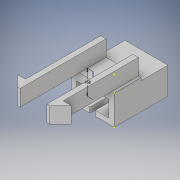
# Autodesk Inventor part: Small USB Cover
Saved by Autodesk Inventor 2018 (Build 220112000, 112)
## iProperties
Created: 2018-01-13
Part Number: Small USB Cover
Material: Generic
Document SubType Name: Modeling
Designer: cruz.anthony
Density: 1 g/cm^3
Appearance: Default
Author: cruz.anthony
Autodesk Inventor part; units mm, degrees
ref_plane "YZ Plane" through (0, 0, 0) normal (1, 0, 0) x (0, 1, 0)
ref_plane "XZ Plane" through (0, 0, 0) normal (0, 1, 0) x (-1, 0, 0)
ref_plane "XY Plane" through (0, 0, 0) normal (0, 0, 1) x (1, 0, 0)
sketch "Sketch1" plane through (0, 0, 0) normal (0, 1, 0) x (-1, 0, 0)
  line L0 (0, 0) -> (20.32, 0)
  line L1 (20.32, 0) -> (20.32, -27.94)
  line L2 (20.32, -27.94) -> (0, -27.94)
  line L3 (0, -27.94) -> (0, 0)
  dimension "d0" = 20.32
  dimension "d1" = 27.94
  constraints: 8 end point, 2 parallel, 1 horizontal, 1 perpendicular
  measures "d0" distance of L1.end L2.end
  measures "d1" distance of L0.end L1.end
extrude "Extrusion1" add sketch "Sketch1" along normal blind 12.7
sketch "Sketch2" plane through (-20.32, 0, 0) normal (0, 0, 1) x (1, 0, 0)
  line L0 (2.54, 2.54) -> (17.78, 2.54)
  line L1 (17.78, 2.54) -> (17.78, 10.16)
  line L2 (17.78, 10.16) -> (2.54, 10.16)
  line L3 (2.54, 10.16) -> (2.54, 2.54)
  point P0 (0, 0)
  dimension "d6" = 15.24
  dimension "d7" = 7.62
  constraints: 8 end point, 2 parallel, 1 horizontal, 1 perpendicular
  measures "d6" distance of L2.end L1.end
  measures "d7" distance of L1.end L0.end
extrude "Extrusion2" cut sketch "Sketch2" against normal blind 22.86
sketch "Sketch3" plane through (0, 0, -27.94) normal (0, 0, -1) x (-1, 0, 0)
  line L0 (0, 0) -> (0, 12.7) projected
  line L1 (0, 0) -> (20.32, 0) projected
  line L2 (0, 12.7) -> (20.32, 12.7)
  line L3 (20.32, 12.7) -> (20.32, 0)
  line L4 (20.32, 0) -> (0, 0)
  line L5 (0, 0) -> (0, 12.7)
  constraints: 8 end point, 2 parallel, 1 horizontal, 1 perpendicular
extrude "Extrusion3" cut sketch "Sketch3" against normal blind 2.54
sketch "Sketch4" plane through (0, 0, 0) normal (0, -1, 0) x (1, 0, 0)
  line L0 (-8.89, 0) -> (-11.43, 0)
  line L1 (-11.43, 0) -> (-11.43, -25.4)
  line L2 (-11.43, -25.4) -> (-8.89, -25.4)
  line L3 (-8.89, -25.4) -> (-8.89, 0)
  line L4 (-20.32, 0) -> (-20.32, -25.4) projected
  line L5 (0, -25.4) -> (0, 0) projected
  dimension "d12" = 8.89
  dimension "d32" = 8.89
  constraints: 8 end point, 2 parallel, 1 horizontal, 1 perpendicular
  measures "d12" distance of L5.end L0.start
  measures "d32" distance between parallel lines of L4 L1
sketch "Sketch5" plane through (0, 0, -25.4) normal (0, 0, -1) x (-1, 0, 0)
  line L0 (0, 0) -> (20.32, 0) projected
  line L1 (10.16, 0) -> (10.16, 6.35)
  circle A0 centre (10.16, 6.35) radius 1.27
  dimension "d14" = 6.35
  dimension "d15" = 2.54
  constraints: 2 end point, 1 centre point, 1 coincident, 1 midpoint, 1 vertical
  measures "d14" distance of L1.start L1.end
  measures "d15" diameter of A0
extrude "Extrusion4" cut sketch "Sketch5" against normal blind 2.54
extrude "Extrusion5" cut sketch "Sketch4" against normal blind 6.35
sketch "Sketch8" plane through (0, 12.7, 0) normal (0, 1, 0) x (1, 0, 0)
  line L0 (0, 25.4) -> (0, 0) projected
  line L1 (-20.32, 0) -> (-20.32, 25.4) projected
  line L2 (0, 0) -> (-20.32, 0)
  line L3 (-20.32, 0) -> (-20.32, 12.7)
  line L4 (-20.32, 12.7) -> (0, 12.7)
  line L5 (0, 12.7) -> (0, 0)
  constraints: 8 end point, 2 parallel, 1 horizontal, 1 midpoint, 1 perpendicular
extrude "Extrusion8" add sketch "Sketch8" along normal blind 2.54
sketch "Sketch9" plane through (-17.78, 10.16, 0) normal (0, 0, 1) x (1, 0, 0)
  arc A0 (8.89, -3.81) -> (6.35, -3.81) centre (7.62, -3.81) ccw projected
  line L0 (7.62, -3.81) -> (7.62, 7.62)
  point P0 (17.78, -10.16)
  dimension "d36" = 11.43
  constraints: 2 end point, 1 vertical
  measures "d36" distance of L0.start L0.end
sketch "Sketch10" plane through (0, 15.24, 0) normal (0, 1, 0) x (1, 0, 0)
  line L0 (-11.43, 0) -> (-20.32, 0) projected
  line L1 (-20.32, 0) -> (0, 0)
  line L2 (0, 0) -> (0, 12.7)
  line L3 (0, 12.7) -> (-20.32, 12.7)
  line L4 (-20.32, 12.7) -> (-20.32, 0)
  constraints: 8 end point, 2 parallel, 1 horizontal, 1 perpendicular
extrude "Extrusion9" cut sketch "Sketch10" against normal blind 1.27
sketch "Sketch11" plane through (0, 13.97, 0) normal (0, 1, 0) x (1, 0, 0)
  point P0 (0, 0)
sketch "Sketch12" plane through (0, 13.97, 0) normal (0, 1, 0) x (1, 0, 0)
  line L0 (-17.78, 0) -> (-2.54, 0) projected
  line L1 (-10.16, 0) -> (-10.16, 12.7099)
  line L2 (-10.16, 0) -> (-16.51, 0)
  line L3 (-11.43, 0) -> (-20.32, 0) projected
  line L4 (-10.16, 0) -> (-3.81, 0)
  line L5 (-3.81, 0) -> (0, 0)
  line L6 (0, 0) -> (0, 12.7099)
  line L7 (0, 12.7099) -> (-3.81, 12.7099)
  line L8 (-3.81, 12.7099) -> (-3.81, 0)
  line L9 (-20.32, 0) -> (-20.32, 12.7) projected
  line L10 (-16.51, 0) -> (-20.32, 0)
  line L11 (-20.32, 0) -> (-20.32, 12.7)
  line L12 (-20.32, 12.7) -> (-16.51, 12.7)
  line L13 (-16.51, 12.7) -> (-16.51, 0)
  dimension "d39" = 6.35
  dimension "d40" = 6.35
  constraints: 22 end point, 4 parallel, 2 horizontal, 2 perpendicular, 2 point on line, 1 midpoint, 1 vertical
  measures "d39" distance of L1.start L2.end
  measures "d40" distance of L1.start L4.end
extrude "Extrusion10" add sketch "Sketch12" along normal blind 7.62
sketch "Sketch13" plane through (-17.78, 10.16, 0) normal (0, 0, 1) x (1, 0, 0)
  line L0 (17.78, 3.81) -> (17.78, 11.43) projected
  line L1 (1.27, 3.81) -> (13.97, 3.81) projected
  line L2 (17.78, 11.43) -> (13.97, 11.43)
  line L3 (13.97, 11.43) -> (13.97, 3.81)
  line L4 (13.97, 3.81) -> (17.78, 3.81)
  line L5 (17.78, 3.81) -> (17.78, 11.43)
  line L6 (1.27, 11.43) -> (-2.54, 11.43) projected
  line L7 (-2.54, 2.54) -> (-2.54, 11.43) projected
  line L8 (1.27, 11.43) -> (-2.54, 11.43)
  line L9 (-2.54, 11.43) -> (-2.54, 3.81)
  line L10 (-2.54, 3.81) -> (1.27, 3.81)
  line L11 (1.27, 3.81) -> (1.27, 11.43)
  point P0 (17.78, -10.16)
  constraints: 16 end point, 4 parallel, 2 horizontal, 2 perpendicular, 1 point on line
extrude "Extrusion11" add sketch "Sketch13" along normal blind 27.94
sketch "Sketch14" plane through (0, 0, 0) normal (1, 0, 0) x (0, 0, -1)
  line L0 (-27.94, 13.97) -> (-27.94, 21.59) projected
  line L1 (12.7, 21.59) -> (-27.94, 21.59) projected
  line L2 (-27.94, 13.97) -> (-22.86, 13.97)
  line L3 (-22.86, 13.97) -> (-22.86, 21.59)
  line L4 (-22.86, 21.59) -> (-27.94, 21.59)
  line L5 (-27.94, 21.59) -> (-27.94, 13.97)
  point P0 (0, 0)
  dimension "d45" = 5.08
  constraints: 8 end point, 2 parallel, 1 horizontal, 1 perpendicular, 1 point on line
  measures "d45" distance of L4.end L3.end
sketch "Sketch15" plane through (0, 21.59, 0) normal (0, 1, 0) x (1, 0, 0)
  point P0 (0, 0)
extrude "Extrusion12" add sketch "Sketch14" along normal blind 2.54
sketch "Sketch16" plane through (-20.32, 0, -25.4) normal (-1, 0, 0) x (0, 0, 1)
  line L0 (48.26, 21.59) -> (53.34, 21.59) projected
  line L1 (53.34, 13.97) -> (48.26, 13.97) projected
  line L2 (53.34, 21.59) -> (48.26, 21.59)
  line L3 (48.26, 21.59) -> (48.26, 13.97)
  line L4 (48.26, 13.97) -> (53.34, 13.97)
  line L5 (53.34, 13.97) -> (53.34, 21.59)
  point P0 (25.4, 0)
  constraints: 8 end point, 2 parallel, 1 horizontal, 1 perpendicular
extrude "Extrusion13" add sketch "Sketch16" along normal blind 2.54
chamfer "Chamfer3" distance 5.08 angle 45 1 edges at (-22.86, 17.78, 27.94)
chamfer "Chamfer4" distance 5.08 angle 45 1 edges at (2.54, 17.78, 27.94)
sketch "Sketch17" plane through (-20.32, 0, -25.4) normal (-1, 0, 0) x (0, 0, 1)
  line L0 (12.7, 12.7) -> (12.7, 21.59) projected
  line L1 (25.4, 13.97) -> (48.26, 13.97) projected
  line L2 (12.7, 21.59) -> (48.26, 21.59)
  line L3 (48.26, 21.59) -> (48.26, 13.97)
  line L4 (48.26, 13.97) -> (12.7, 13.97)
  line L5 (12.7, 13.97) -> (12.7, 21.59)
  point P0 (25.4, 0)
  constraints: 8 end point, 2 parallel, 1 horizontal, 1 perpendicular
extrude "Extrusion14" cut sketch "Sketch17" against normal blind 1.27
sketch "Sketch18" plane through (0, 0, 0) normal (1, 0, 0) x (0, 0, -1)
  line L0 (12.7099, 13.97) -> (12.7099, 21.59) projected
  line L1 (0, 13.97) -> (-22.86, 13.97) projected
  line L2 (12.7099, 21.59) -> (-22.86, 21.59)
  line L3 (-22.86, 21.59) -> (-22.86, 13.97)
  line L4 (-22.86, 13.97) -> (12.7099, 13.97)
  line L5 (12.7099, 13.97) -> (12.7099, 21.59)
  point P0 (0, 0)
  constraints: 8 end point, 2 parallel, 1 horizontal, 1 perpendicular
extrude "Extrusion15" cut sketch "Sketch18" against normal blind 1.27
body "Solid1"
